Autodesk Inventor part; units mm, degrees
(part 2 of 2)
sketch "Sketch7" plane through (-15, -11.125, -16.5) normal (0, -1, 0) x (1, 0, 0)
  line L0 (30, 0) -> (30, 33) projected
  line L1 (30, 1.4) -> (28.5717, 0)
  line L2 (28.5717, 0) -> (35.5717, -7.1414)
  line L3 (35.5717, -7.1414) -> (37, -5.7414)
  line L4 (37, -5.7414) -> (30, 1.4)
  line L5 (0, 0) -> (30, 0) projected
  circle A0 centre (36.2859, -6.4414) radius 5
  line L6 (15, 0) -> (15, 33)
  line L7 (30, 33) -> (0, 33) projected
  line L8 (30, 16.5) -> (0, 16.5)
  line L9 (0, 33) -> (0, 0) projected
  line L10 (0, 1.4) -> (1.4283, 0)
  line L11 (1.4283, 0) -> (-5.5717, -7.1414)
  line L12 (-5.5717, -7.1414) -> (-7, -5.7414)
  line L13 (-7, -5.7414) -> (0, 1.4)
  circle A1 centre (-6.2859, -6.4414) radius 5
  line L14 (30, 31.6) -> (28.5717, 33)
  line L15 (28.5717, 33) -> (35.5717, 40.1414)
  line L16 (35.5717, 40.1414) -> (37, 38.7414)
  line L17 (37, 38.7414) -> (30, 31.6)
  circle A2 centre (36.2859, 39.4414) radius 5
  line L18 (1.4283, 33) -> (-5.5717, 40.1414)
  line L19 (-7, 38.7414) -> (0, 31.6)
  circle A3 centre (-6.2859, 39.4414) radius 5
  line L20 (-5.5717, 40.1414) -> (-7, 38.7414)
  line L21 (0, 31.6) -> (1.4283, 33)
  point P0 (15, 16.5)
  point P1 (33.5707, 35.2429)
  point P2 (32.1424, 36.6429)
  point P3 (-2.1424, 36.6429)
  point P4 (-3.5707, 35.2429)
  point P5 (-3.5707, -2.2429)
  point P6 (-2.1424, -3.6429)
  point P7 (33.5707, -2.2429)
  point P8 (32.1424, -3.6429)
  dimension "d48" = 2
  dimension "d50" = 1.4
  dimension "d51" = 10
  dimension "d54" = 10
  constraints: 36 end point, 15 symmetric about line, 5 midpoint, 4 centre point, 2 parallel, 2 point on line, 1 perpendicular, 3 other
  measures "d48" distance of L1.start L1.end
  measures "d50" distance of L0.start L1.start
  measures "d51" diameter of A0
  measures "d54" distance of L3.end L1.start
extrude "Micky mouse ears" add sketch "Sketch7" against normal blind 0.25 contours L5 L1 L0 | L0 L4 A0 L2 L5 | A0 L2 L3 L4 | L4 L3 L2 A0 | L14 L7 L0 | L0 L7 L15 A2 L17 | L11 A1 L13 L9 L5 | L5 L9 L10 | A2 L15 L16 L17 | L17 L16 L15 A2 | A1 L13 L12 L11 | L11 L12 L13 A1 | L21 L9 L7 | L7 L9 L19 A3 L18 | A3 L19 L20 L18 | L18 L20 L19 A3
equation "\"d50\" = d49"
equation "\"d49\" = 1.4"
body "Solid1"
